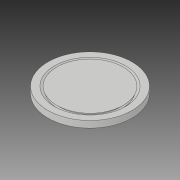
# Autodesk Inventor part: button_test
Saved by Autodesk Inventor 2019.3 (Build 233278000, 278)
## iProperties
Created: 2019-03-01
Part Number: button_test
Material: Generic
Document SubType Name: Modeling
Designer: WW
Density: 1 g/cm^3
Appearance: Default
Author: WW
Autodesk Inventor part; units mm, degrees
ref_plane "YZ Plane" through (0, 0, 0) normal (1, 0, 0) x (0, 1, 0)
ref_plane "XZ Plane" through (0, 0, 0) normal (0, 1, 0) x (-1, 0, 0)
ref_plane "XY Plane" through (0, 0, 0) normal (0, 0, 1) x (1, 0, 0)
sketch "Sketch1" plane through (0, 0, 0) normal (0, 0, 1) x (1, 0, 0)
  line L0 (0, 0) -> (0, -11.2698) construction
  line L1 (0, 0) -> (15, 0)
  line L2 (15, 0) -> (13.5, 1.5)
  line L3 (13.5, 1.5) -> (15, 3)
  line L4 (15, 3) -> (0, 3)
  line L5 (0, 3) -> (0, 0)
  line L6 (15.9899, 3) -> (14.4899, 1.5)
  line L7 (14.4899, 1.5) -> (15.9899, 0)
  line L8 (15.9899, 3) -> (19, 3)
  line L9 (19, 3) -> (19, 0)
  line L10 (19, 0) -> (15.9899, 0)
  point P0 (0, 1.5)
  dimension "d0" = 3
  dimension "d1" = 30
  dimension "d2" = 45
  dimension "d3" = 0.7
  dimension "d6" = 38
  constraints: 22 end point, 4 perpendicular, 3 horizontal alignment, 2 horizontal, 2 vertical, 1 midpoint, 1 parallel, 1 other
  measures "d0" distance between parallel lines of L1 L4
  measures "d1" diameter of L1.end L0
  measures "d2" angle of L4 L3
  measures "d3" distance between parallel lines of L3 L6
  measures "d6" diameter of L9 L0
revolve "Revolution1" add sketch "Sketch1" angle 360 about axis through (0, 0, 0) along (0, -1, 0)
body "Solid1"
